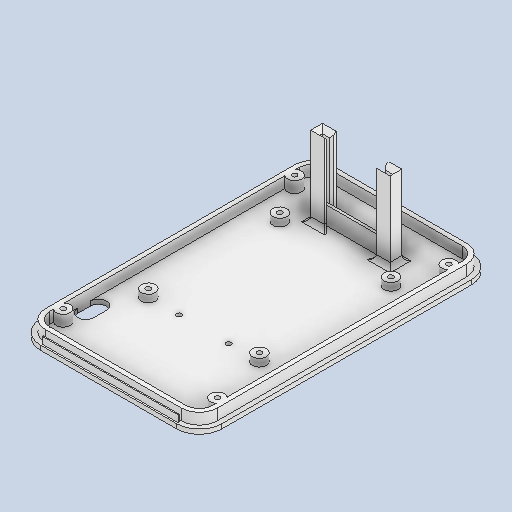
# Autodesk Inventor part: BOTTOM
Saved by Autodesk Inventor 2023 (Build 270158000, 158)
## iProperties
Created: 2023-03-14
Part Number: BOTTOM
Material: Generic
Document SubType Name: Modeling
Designer: Amos Yu
Density: 1 g/cm^3
Appearance: White
Author: Amos Yu
Autodesk Inventor part; units mm, degrees
ref_plane "YZ Plane" through (0, 0, 0) normal (1, 0, 0) x (0, 1, 0)
ref_plane "XZ Plane" through (0, 0, 0) normal (0, 1, 0) x (-1, 0, 0)
ref_plane "XY Plane" through (0, 0, 0) normal (0, 0, 1) x (1, 0, 0)
sketch "Sketch1" plane through (0, 0, 0) normal (0, 1, 0) x (-1, 0, 0)
  line L0 (-10, 0) -> (-70, 0)
  line L1 (-80, -10) -> (-80, -120)
  line L2 (-70, -130) -> (-10, -130)
  line L3 (0, -120) -> (0, -10)
  arc A0 (-80, -120) -> (-70, -130) centre (-70, -120) ccw
  arc A1 (-10, -130) -> (0, -120) centre (-10, -120) ccw
  arc A2 (-70, 0) -> (-80, -10) centre (-70, -10) ccw
  arc A3 (0, -10) -> (-10, 0) centre (-10, -10) ccw
  point P0 (0, 0)
  point P1 (-80, -130)
  point P2 (-80, 0)
  point P3 (0, -130)
  dimension "d0" = 80
  dimension "d1" = 130
  dimension "d4" = 10
  constraints: 8 end point, 8 point on circle, 8 point on line, 8 tangent, 4 centre point, 3 equal radius, 2 parallel, 1 horizontal, 1 perpendicular
  measures "d0" distance of point (0, -130) point (-80, -130)
  measures "d1" distance of point (-80, -130) point (-80, 0)
  measures "d4" radius of A0
extrude "Extrusion1" add sketch "Sketch1" along normal blind 2
sketch "Sketch3" plane through (0, 2, 0) normal (0, 1, 0) x (1, 0, 0)
  line L0 (0, 120) -> (0, 10) projected
  line L1 (70, 130) -> (10, 130) projected
  line L2 (80, 10) -> (80, 120) projected
  line L3 (10, 0) -> (70, 0) projected
  line L4 (10, 127.9) -> (70, 127.9)
  line L5 (77.9, 120) -> (77.9, 10)
  line L6 (70, 2.1) -> (10, 2.1)
  line L7 (2.1, 10) -> (2.1, 120)
  arc A0 (10, 130) -> (0, 120) centre (10, 120) ccw projected
  arc A1 (80, 120) -> (0, 120) centre (70, 120) ccw projected
  arc A2 (0, 10) -> (80, 10) centre (70, 10) ccw projected
  arc A3 (0, 10) -> (10, 0) centre (10, 10) ccw projected
  arc A4 (10, 127.9) -> (2.1, 120) centre (10, 120) ccw
  arc A5 (77.9, 120) -> (70, 127.9) centre (70, 120) ccw
  arc A6 (70, 2.1) -> (77.9, 10) centre (70, 10) ccw
  arc A7 (2.1, 10) -> (10, 2.1) centre (10, 10) ccw
  line L8 (10, 4.1) -> (70, 4.1)
  arc A8 (70, 4.1) -> (75.9, 10) centre (70, 10) ccw
  line L9 (75.9, 10) -> (75.9, 120)
  arc A9 (75.9, 120) -> (70, 125.9) centre (70, 120) ccw
  line L10 (70, 125.9) -> (10, 125.9)
  arc A10 (10, 125.9) -> (4.1, 120) centre (10, 120) ccw
  line L11 (4.1, 120) -> (4.1, 10)
  arc A11 (4.1, 10) -> (10, 4.1) centre (10, 10) ccw
  point P0 (0, 0)
  dimension "d11" = 2.1
  dimension "d12" = 2.1
  dimension "d13" = 2.1
  dimension "d14" = 2.1
  dimension "d15" = 7.9
  dimension "d16" = 2
  constraints: 16 end point, 16 point on circle, 8 centre point, 8 tangent, 4 parallel, 3 equal radius, 2 perpendicular, 1 horizontal, 9 other
  measures "d11" distance between parallel lines of L2 L5
  measures "d12" distance between parallel lines of L0 L7
  measures "d13" distance between parallel lines of L6 L3
  measures "d14" distance between parallel lines of L1 L4
  measures "d15" radius of A4
  measures "d16" distance between parallel lines of L6 L8
extrude "Extrusion2" add sketch "Sketch3" along normal blind 4.9 contours A4 A1 | A1 A4 L4 A5 L5 A6 L6 A7 L7 | A5 A1
sketch "Sketch4" plane through (0, 2, 0) normal (0, 1, 0) x (1, 0, 0)
  circle A0 centre (6, 14) radius 3.1
  circle A1 centre (6, 14) radius 1.1
  line L0 (0, 120) -> (0, 10) projected
  line L1 (10, 0) -> (70, 0) projected
  circle A2 centre (6, 116) radius 3.1
  circle A3 centre (6, 116) radius 1.1
  circle A4 centre (74, 14) radius 3.1
  circle A5 centre (74, 14) radius 1.1
  circle A6 centre (74, 116) radius 3.1
  circle A7 centre (74, 116) radius 1.1
  circle A8 centre (15.5, 42) radius 1.1
  circle A9 centre (15.5, 42) radius 3.1
  circle A10 centre (15.5, 100) radius 1.1
  circle A11 centre (15.5, 100) radius 3.1
  circle A12 centre (64.5, 42) radius 1.1
  circle A13 centre (64.5, 42) radius 3.1
  circle A14 centre (64.5, 100) radius 1.1
  circle A15 centre (64.5, 100) radius 3.1
  line L2 (15.5, 42) -> (64.5, 42) construction
  point P0 (0, 0)
  point P1 (40, 42)
  point P2 (40, 0)
  dimension "d20" = 2.2
  dimension "d21" = 14
  dimension "d22" = 6
  dimension "d25" = 102
  dimension "d28" = 68
  dimension "d35" = 2
  dimension "d59" = 2.2
  dimension "d60" = 2
  dimension "d63" = 58
  dimension "d66" = 49
  dimension "d69" = 42
  constraints: 16 centre point, 8 coincident, 3 horizontal, 2 end point, 2 midpoint, 2 vertical, 1 vertical alignment, 24 other
  measures "d20" diameter of A1
  measures "d21" vertical distance of point (0, 0) A0.centre
  measures "d22" horizontal distance of point (0, 0) A0.centre
  measures "d25" distance of A0.centre A2.centre
  measures "d28" distance of A0.centre A4.centre
  measures "d35" radial gap between concentric circles of A1 A0
  measures "d59" diameter of A8
  measures "d60" radial gap between concentric circles of A8 A9
  measures "d63" distance of A8.centre A10.centre
  measures "d66" distance of A8.centre A12.centre
  measures "d69" vertical distance of point (0, 0) A8.centre
extrude "Extrusion3" add sketch "Sketch4" along normal blind 4.9 contours A0 | A2 | A4 | A6
extrude "Extrusion4" cut sketch "Sketch4" along normal blind 4.9 contours A1 | A3 | A5 | A7 | A8 | A10 | A12 | A14
sketch "Sketch5" plane through (0, 0, 0) normal (0, -1, 0) x (1, 0, 0)
  circle A0 centre (6, -14) radius 2.1
  line L0 (0, -120) -> (0, -10) projected
  line L1 (10, 0) -> (70, 0) projected
  circle A1 centre (74, -14) radius 2.1
  circle A2 centre (6, -116) radius 2.1
  circle A3 centre (74, -116) radius 2.1
  circle A4 centre (15.5, -42) radius 2.1
  circle A5 centre (15.5, -100) radius 2.1
  circle A6 centre (64.5, -42) radius 2.1
  circle A7 centre (64.5, -100) radius 2.1
  line L2 (15.5, -42) -> (64.5, -42) construction
  point P0 (0, 0)
  point P1 (40, -42)
  point P2 (40, 0)
  dimension "d36" = 4.2
  dimension "d37" = 14
  dimension "d38" = 6
  dimension "d41" = 68
  dimension "d44" = 102
  dimension "d49" = 4.2
  dimension "d52" = 58
  dimension "d55" = 49
  dimension "d58" = 42
  constraints: 8 centre point, 3 horizontal, 2 end point, 2 midpoint, 2 vertical, 1 vertical alignment, 12 other
  measures "d36" diameter of A0
  measures "d37" vertical distance of point (0, 0) A0.centre
  measures "d38" horizontal distance of point (0, 0) A0.centre
  measures "d41" distance of A0.centre A1.centre
  measures "d44" distance of A0.centre A2.centre
  measures "d49" diameter of A4
  measures "d52" distance of L2.start A5.centre
  measures "d55" distance of L2.start L2.end
  measures "d58" vertical distance of point (0, 0) L2.start
extrude "Extrusion5" cut sketch "Sketch5" against normal blind 2.1
extrude "Extrusion6" add sketch "Sketch4" along normal blind 3.3 contours A9 | A11 | A13 | A15
sketch "Sketch6" plane through (0, 2, 0) normal (0, 1, 0) x (1, 0, 0)
  circle A0 centre (29, 42) radius 1.1
  circle A1 centre (51, 42) radius 1.1
  line L0 (29, 42) -> (51, 42) construction
  line L1 (10, 0) -> (70, 0) construction
  point P0 (0, 0)
  point P1 (40, 42)
  point P2 (40, 0)
  dimension "d72" = 2.2
  dimension "d73" = 2.2
  dimension "d74" = 22
  dimension "d75" = 42
  constraints: 2 centre point, 2 end point, 2 midpoint, 1 horizontal, 1 horizontal alignment, 1 vertical alignment
  measures "d72" diameter of A0
  measures "d73" diameter of A1
  measures "d74" distance of L0.end L0.start
  measures "d75" vertical distance of point (0, 0) L0.start
extrude "Extrusion8" cut sketch "Sketch6" against normal up to surface (2 mm away)
sketch "Sketch7" plane through (0, 2, 0) normal (0, 1, 0) x (1, 0, 0)
  line L0 (24.5, 109.8) -> (27.5, 109.8)
  line L1 (27.5, 109.8) -> (28.5, 110.8)
  line L2 (28.5, 110.8) -> (28.5, 111.8)
  line L3 (28.5, 111.8) -> (22.5, 111.8)
  line L4 (22.5, 111.8) -> (22.5, 106.6)
  line L5 (22.5, 106.6) -> (28.5, 106.6)
  line L6 (27.5, 108.6) -> (28.5, 107.6)
  line L7 (28.5, 107.6) -> (28.5, 106.6)
  line L8 (24.5, 108.6) -> (27.5, 108.6)
  line L9 (40, 111.8) -> (40, 106.6) construction
  line L10 (24.5, 109.8) -> (24.5, 108.6)
  line L11 (55.5, 109.8) -> (52.5, 109.8)
  line L12 (52.5, 109.8) -> (51.5, 110.8)
  line L13 (51.5, 110.8) -> (51.5, 111.8)
  line L14 (51.5, 111.8) -> (57.5, 111.8)
  line L15 (57.5, 111.8) -> (57.5, 106.6)
  line L16 (57.5, 106.6) -> (51.5, 106.6)
  line L17 (52.5, 108.6) -> (51.5, 107.6)
  line L18 (51.5, 107.6) -> (51.5, 106.6)
  line L19 (55.5, 108.6) -> (52.5, 108.6)
  line L20 (55.5, 109.8) -> (55.5, 108.6)
  line L21 (27.5, 109.8) -> (52.5, 109.8)
  line L22 (52.5, 108.6) -> (27.5, 108.6)
  line L23 (70, 130) -> (10, 130) projected
  point P0 (0, 0)
  point P1 (40, 130)
  dimension "d84" = 1
  dimension "d89" = 1
  dimension "d90" = 2
  dimension "d91" = 2
  dimension "d92" = 2
  dimension "d93" = 31
  dimension "d94" = 1.2
  dimension "d95" = 135
  dimension "d96" = 135
  dimension "d97" = 21.4
  dimension "d104" = 4
  constraints: 46 end point, 10 symmetric about line, 4 vertical, 2 horizontal alignment, 2 perpendicular, 2 vertical alignment, 1 collinear, 1 horizontal, 1 midpoint, 1 parallel
  measures "d84" distance of L1.end L2.end
  measures "d89" distance of L6.end L5.end
  measures "d90" distance between parallel lines of L4 L10
  measures "d91" distance between parallel lines of L8 L5
  measures "d92" distance between parallel lines of L3 L0
  measures "d93" distance between parallel lines of L20 L10
  measures "d94" distance between parallel lines of L0 L8
  measures "d95" angle of L7 L6
  measures "d96" angle of L2 L1
  measures "d97" distance between parallel lines of L23 L22
  measures "d104" horizontal distance of L0.start L1.end
extrude "Extrusion9" add sketch "Sketch7" along normal blind 35 contours L10 L8 L6 L7 L5 L4 L3 L2 L1 L0 | L12 L13 L14 L15 L16 L18 L17 L19 L20 L11
extrude "Extrusion10" add sketch "Sketch7" along normal blind 7.9 contours L0 L21 L11 L20 L19 L22 L8 L10
sketch "Sketch8" plane through (0, 37, 0) normal (0, 1, 0) x (1, 0, 0)
  line L0 (22.5, 106.6) -> (57.5, 106.6)
  line L1 (57.5, 106.6) -> (57.5, 111.8)
  line L2 (57.5, 111.8) -> (22.5, 111.8)
  line L3 (22.5, 111.8) -> (22.5, 106.6)
  point P0 (0, 0)
  constraints: 8 end point, 2 coincident, 2 parallel, 1 horizontal, 1 perpendicular
extrude "Extrusion11" cut sketch "Sketch8" against normal blind 2 draft -45
fillet "Fillet1" radius 2 10 edges at (57.5, 2, -109.2) (22.5, 2, -109.2) (25.5, 2, -106.6) (54.5, 2, -106.6) (54.5, 2, -111.8) (25.5, 2, -111.8) (28.5, 2, -111.3) (28.5, 2, -107.1) (51.5, 2, -107.1) (51.5, 2, -111.3)
sketch "Sketch9" plane through (0, 2, 0) normal (0, 1, 0) x (1, 0, 0)
  line L0 (10.2, 1.2) -> (70, 1.2)
  line L1 (70, 1.2) -> (70, 0.7)
  line L2 (70, 0.7) -> (10.2, 0.7)
  line L3 (10.2, 0.7) -> (10.2, 1.2)
  line L4 (80, 10) -> (80, 120) projected
  line L5 (10, 2.1) -> (70, 2.1) projected
  line L6 (10, 0) -> (70, 0) construction
  point P0 (0, 0)
  dimension "d106" = 0.5
  dimension "d107" = 10.2
  dimension "d108" = 10
  dimension "d109" = 0.7
  constraints: 8 end point, 2 parallel, 1 horizontal, 1 perpendicular
  measures "d106" distance of L2.end L0.start
  measures "d107" distance from line of point (0, 0) L3
  measures "d108" distance between parallel lines of L4 L1
  measures "d109" distance between parallel lines of L6 L2
extrude "Extrusion12" add sketch "Sketch9" along normal blind 3
sketch "Sketch10" plane through (0, 2, 0) normal (0, 1, 0) x (1, 0, 0)
  line L0 (7.7, 27.75) -> (7.7, 22.25) construction
  line L1 (4.1, 27.75) -> (4.1, 22.25)
  line L2 (11.3, 22.25) -> (11.3, 27.75)
  arc A0 (11.3, 27.75) -> (4.1, 27.75) centre (7.7, 27.75) ccw
  arc A1 (4.1, 22.25) -> (11.3, 22.25) centre (7.7, 22.25) ccw
  line L3 (4.1, 16.4495) -> (4.1, 113.5505) construction
  point P0 (0, 0)
  point P1 (7.7, 25)
  point P2 (7.7, 31.35)
  point P3 (7.7, 18.65)
  dimension "d112" = 12.7
  dimension "d113" = 7.2
  dimension "d117" = 25
  constraints: 8 end point, 6 point on circle, 4 tangent, 2 centre point, 1 collinear, 1 midpoint, 1 parallel, 1 vertical
  measures "d112" distance of point (7.7, 31.35) point (7.7, 18.65)
  measures "d113" distance between parallel lines of L2 L1
  measures "d117" vertical distance of point (7.7, 25) point (0, 0)
extrude "Extrusion13" cut sketch "Sketch10" against normal up to surface (2 mm away)
equation "\"d0\" = total_width"
equation "\"d1\" = total_depth"
equation "\"d4\" = fillet_outer_radius"
equation "\"d2\" = thickness"
equation "\"d11\" = thickness + tol"
equation "\"d12\" = thickness + tol"
equation "\"d13\" = thickness + tol"
equation "\"d14\" = thickness + tol"
equation "\"d15\" = -thickness + fillet_outer_radius - tol"
equation "\"d16\" = thickness"
equation "\"d17\" = lip_height - tol"
equation "\"d20\" = bolt_thread_diameter + 2 * tol"
equation "\"d21\" = bolt_inset_depth"
equation "\"d22\" = bolt_inset_width"
equation "\"d25\" = total_depth - 2 * bolt_inset_depth"
equation "\"d28\" = total_width - 2 * bolt_inset_width"
equation "\"d35\" = thickness"
equation "\"d59\" = bolt_thread_diameter + 2 * tol"
equation "\"d60\" = thickness"
equation "\"d63\" = pi_mount_depth"
equation "\"d66\" = pi_mount_width"
equation "\"d69\" = pi_mount_inset_depth"
equation "\"d31\" = lip_height - tol"
equation "\"d33\" = lip_height - tol"
equation "\"d36\" = bolt_head_diameter + 2 * tol"
equation "\"d37\" = bolt_inset_depth"
equation "\"d38\" = bolt_inset_width"
equation "\"d41\" = total_width - 2 * bolt_inset_width"
equation "\"d44\" = total_depth - 2 * bolt_inset_depth"
equation "\"d49\" = bolt_head_diameter + 2 * tol"
equation "\"d52\" = pi_mount_depth"
equation "\"d55\" = pi_mount_width"
equation "\"d58\" = pi_mount_inset_depth"
equation "\"d47\" = bolt_head_height + tol"
equation "\"d70\" = -tol + lip_height - pi_board_height"
equation "\"d72\" = bolt_thread_diameter + 2 * tol"
equation "\"d73\" = bolt_thread_diameter + 2 * tol"
equation "\"d74\" = clamp_mount_width"
equation "\"d75\" = clamp_mount_inset_depth"
equation "\"d78\" = -tol + lip_height - pi_board_height"
equation "\"d84\" = 0.5 * thickness"
equation "\"d89\" = 0.5 * thickness"
equation "\"d90\" = thickness"
equation "\"d91\" = thickness"
equation "\"d92\" = thickness"
equation "\"d93\" = camera_width + 2 * tol"
equation "\"d94\" = camera_board_depth + 2 * tol"
equation "\"d97\" = camera_depth"
equation "\"d104\" = camera_mount_inset_width"
equation "\"d98\" = camera_mount_height"
equation "\"d100\" = -0.5 * camera_height + 0.5 * total_height - thickness - tol"
equation "\"d102\" = thickness"
equation "\"d105\" = thickness"
equation "\"pi_mount_width\" = 49"
equation "\"pi_mount_depth\" = 58"
equation "\"pi_mount_inset_depth\" = 42"
equation "\"clamp_mount_width\" = 22"
equation "\"clamp_mount_inset_depth\" = 42"
equation "\"pi_board_height\" = 1.6"
equation "\"camera_depth\" = 21.4"
equation "\"camera_width\" = 30.8"
equation "\"camera_board_depth\" = 1"
equation "\"camera_mount_inset_width\" = 4"
equation "\"camera_mount_height\" = 35"
equation "\"camera_height\" = 25"
equation "\"usbc_hole_depth\" = 12.5"
equation "\"usbc_hole_width\" = 7"
equation "\"fillet_outer_radius\" = 10"
equation "\"thickness\" = 2"
equation "\"tol\" = 0.1"
equation "\"lip_height\" = 5"
equation "\"bolt_thread_diameter\" = 2"
equation "\"total_depth\" = 130"
equation "\"bolt_inset_depth\" = 14"
equation "\"total_width\" = 80"
equation "\"bolt_inset_width\" = 6"
equation "\"bolt_head_diameter\" = 4"
equation "\"bolt_head_height\" = 2"
equation "\"total_height\" = 45"
body "Solid1"
